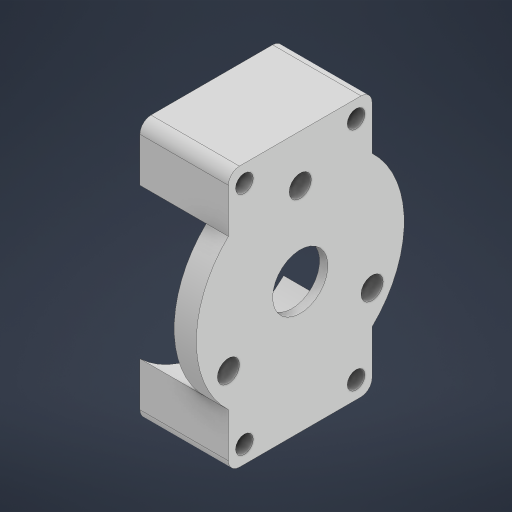
# Autodesk Inventor part: MotorMount_sub
Saved by Autodesk Inventor 2024.2 (Build 282272000, 272)
## iProperties
Created: 2023-12-20
Part Number: MotorMount_sub
Material: 一般
Document SubType Name: Modeling
Designer: Hanaoka
Density: 1 g/cm^3
Appearance: 既定
Author: Hanaoka
Autodesk Inventor part; units mm, degrees
ref_plane "YZ Plane" through (0, 0, 0) normal (1, 0, 0) x (0, 1, 0)
ref_plane "XZ Plane" through (0, 0, 0) normal (0, 1, 0) x (-1, 0, 0)
ref_plane "XY Plane" through (0, 0, 0) normal (0, 0, 1) x (1, 0, 0)
derived "0_3.ipt"
sketch "スケッチ1" plane through (0, 0, 0) normal (-1, 0, 0) x (0, 0, 1)
  circle A0 centre (0, 0) radius 9.4 projected
  circle A1 centre (8.0839, 3.3485) radius 0.4 construction
  circle A2 centre (-3.75, -6.4952) radius 1 construction
  circle A3 centre (7.5, 0) radius 1 construction
  circle A4 centre (-3.75, 6.4952) radius 1 construction
  circle A5 centre (0, 0) radius 6 projected
  circle A6 centre (0, 0) radius 2.5
  circle A7 centre (0, 7.5) radius 1
  circle A8 centre (0, 0) radius 7.5 construction
  line L0 (0, -13.16) -> (0, 13.16) projected
  circle A9 centre (-6.4952, -3.75) radius 1
  circle A10 centre (6.4952, -3.75) radius 1
  dimension "d3" = 5
  dimension "d26" = 360
  constraints: 5 centre point, 2 coincident, 2 point on circle, 1 equal radius, 1 point on line, 7 other
  measures "d3" diameter of A6
extrude "押し出し1" add sketch "スケッチ1" against normal blind 2 contours A0 L0 A5 A7 | L0 A7 A5 A0 | L0 A6 A5 | A5 L0 A6
extrude "押し出し2" cut sketch "スケッチ1" against normal blind 1.25 contours L0 A6 A5 | A5 L0 A6
sketch "スケッチ4" plane through (2, 0, 0) normal (1, 0, 0) x (0, 0, -1)
  circle A0 centre (0, 0) radius 9.4 projected
  line L0 (-6.5, 6.7904) -> (-6.5, 10.7904)
  line L1 (-5.5, 11.7904) -> (5.5, 11.7904)
  line L2 (6.5, 10.7904) -> (6.5, 6.7904)
  line L3 (-6.5, -6.7904) -> (-6.5, -10.7904)
  line L4 (-5.5, -11.7904) -> (5.5, -11.7904)
  line L5 (6.5, -10.7904) -> (6.5, -6.7904)
  arc A1 (-5.5, 11.7904) -> (-6.5, 10.7904) centre (-5.5, 10.7904) ccw
  arc A2 (6.5, 10.7904) -> (5.5, 11.7904) centre (5.5, 10.7904) ccw
  arc A3 (5.5, -11.7904) -> (6.5, -10.7904) centre (5.5, -10.7904) ccw
  arc A4 (-6.5, -10.7904) -> (-5.5, -11.7904) centre (-5.5, -10.7904) ccw
  circle A5 centre (0, 0) radius 14 construction
  circle A6 centre (5.05, 10.2204) radius 0.8
  circle A7 centre (5.05, 10.2204) radius 2 construction
  circle A8 centre (0, 0) radius 9.4 projected
  circle A9 centre (-5.05, 10.2204) radius 0.8
  circle A10 centre (-5.05, 10.2204) radius 2 construction
  line L6 (-5.05, 10.2204) -> (-5.05, 7.9283) construction
  line L7 (5.05, 10.2204) -> (5.05, 7.9283) construction
  circle A11 centre (5.05, -10.2204) radius 2 construction
  circle A12 centre (5.05, -10.2204) radius 0.8
  circle A13 centre (-5.05, -10.2204) radius 0.8
  circle A14 centre (-5.05, -10.2204) radius 2 construction
  point P0 (-6.5, -11.7904)
  point P1 (6.5, -11.7904)
  dimension "d8" = 1
  dimension "d9" = 28
  dimension "d13" = 4
  dimension "d14" = 11
  dimension "d15" = 1.6
  dimension "d16" = 4
  dimension "d17" = 8.5
  dimension "d20" = 360
  constraints: 16 end point, 14 point on circle, 13 centre point, 10 tangent, 8 point on line, 5 coincident, 5 equal radius, 3 equal length, 3 perpendicular, 2 vertical, 1 parallel, 17 other
  measures "d8" radius of A1
  measures "d9" diameter of A5
  measures "d13" distance of L2.start L2.end
  measures "d14" distance of L1.start L1.end
  measures "d15" diameter of A6
  measures "d16" diameter of A7
extrude "押し出し3" add sketch "スケッチ4" against normal blind 8 contours A0 L0 A1 L1 A2 L2 | L5 A3 L4 A4 L3 A0
